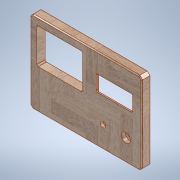
# Autodesk Inventor part: EW_Holzplatte
Saved by Autodesk Inventor 2020 (Build 240168000, 168)
## iProperties
Created: 2020-06-21
Part Number: EW_Holzplatte
Material: Eiche, Rot
Document SubType Name: Modeling
Designer: Johannes
Density: 0.673 g/cm^3
Appearance: Eiche - Fischgrätmuster
Author: Johannes
Autodesk Inventor part; units mm, degrees
ref_plane "YZ Plane" through (0, 0, 0) normal (1, 0, 0) x (0, 1, 0)
ref_plane "XZ Plane" through (0, 0, 0) normal (0, 1, 0) x (-1, 0, 0)
ref_plane "XY Plane" through (0, 0, 0) normal (0, 0, 1) x (1, 0, 0)
sketch "Skizze1" plane through (0, 0, 0) normal (0, 0, 1) x (1, 0, 0)
  line L0 (-122.5, 90) -> (122.5, 90)
  line L1 (122.5, 90) -> (122.5, -90)
  line L2 (122.5, -90) -> (-122.5, -90)
  line L3 (-122.5, -90) -> (-122.5, 90)
  line L4 (-122.5, 90) -> (122.5, -90) construction
  line L5 (122.5, 90) -> (-122.5, -90) construction
  point P0 (0, 0)
  dimension "d0" = 245
  dimension "d1" = 180
  constraints: 12 end point, 2 midpoint, 2 parallel, 1 horizontal, 1 perpendicular
  measures "d0" distance of L1.end L2.end
  measures "d1" distance of L0.end L1.end
extrude "Extrusion1" add sketch "Skizze1" along normal blind 18
sketch "Skizze3" plane through (0, 0, 18) normal (0, 0, 1) x (1, 0, 0)
  line L0 (22.5, 47.5) -> (102.5, 47.5)
  line L1 (102.5, 47.5) -> (102.5, 12.5)
  line L2 (102.5, 12.5) -> (22.5, 12.5)
  line L3 (22.5, 12.5) -> (22.5, 47.5)
  line L4 (22.5, 47.5) -> (102.5, 12.5) construction
  line L5 (102.5, 47.5) -> (22.5, 12.5) construction
  line L6 (122.5, 90) -> (-122.5, 90) projected
  line L7 (122.5, -90) -> (122.5, 90) projected
  point P0 (0, 0)
  point P1 (62.5, 30)
  dimension "d12" = 80
  dimension "d13" = 35
  dimension "d32" = 60
  dimension "d33" = 60
  constraints: 12 end point, 2 midpoint, 2 parallel, 1 horizontal, 1 perpendicular
  measures "d12" distance of L0.start L0.end
  measures "d13" distance of L2.end L0.start
  measures "d32" distance from line of L6 point (62.5, 30)
  measures "d33" distance from line of L7 point (62.5, 30)
extrude "Extrusion2" cut sketch "Skizze3" against normal blind 3
sketch "Skizze4" plane through (0, 0, 0) normal (0, 0, -1) x (-1, 0, 0)
  line L0 (-115, 71.75) -> (-10, 71.75)
  line L1 (-10, 71.75) -> (-10, -25.25)
  line L2 (-10, -25.25) -> (-115, -25.25)
  line L3 (-115, -25.25) -> (-115, 71.75)
  line L4 (-115, 71.75) -> (-10, -25.25) construction
  line L5 (-10, 71.75) -> (-115, -25.25) construction
  line L6 (-122.5, 90) -> (122.5, 90) projected
  line L7 (-122.5, -90) -> (-122.5, 90) projected
  point P0 (0, 0)
  point P1 (-62.5, 23.25)
  dimension "d20" = 60
  dimension "d21" = 105
  dimension "d22" = 97
  dimension "d23" = 18.25
  constraints: 12 end point, 2 midpoint, 2 parallel, 1 horizontal, 1 perpendicular
  measures "d20" distance from line of L7 point (-62.5, 23.25)
  measures "d21" distance of L0.start L0.end
  measures "d22" distance of L2.end L0.start
  measures "d23" distance between parallel lines of L0 L6
extrude "Extrusion3" cut sketch "Skizze4" against normal blind 6
sketch "Skizze5" plane through (0, 0, 6) normal (0, 0, -1) x (-1, 0, 0)
  line L0 (-115, 51) -> (-10, 51)
  line L1 (-10, 51) -> (-10, -5)
  line L2 (-10, -5) -> (-115, -5)
  line L3 (-115, -5) -> (-115, 51)
  line L4 (-115, 51) -> (-10, -5) construction
  line L5 (-10, 51) -> (-115, -5) construction
  line L6 (-122.5, 90) -> (122.5, 90) projected
  line L7 (-122.5, -90) -> (-122.5, 90) projected
  point P0 (0, 0)
  point P1 (-62.5, 23)
  dimension "d26" = 105
  dimension "d34" = 60
  dimension "d35" = 39
  dimension "d36" = 95
  constraints: 12 end point, 2 midpoint, 2 parallel, 1 horizontal, 1 perpendicular
  measures "d26" distance of L0.start L0.end
  measures "d34" distance from line of L7 point (-62.5, 23)
  measures "d35" distance between parallel lines of L6 L0
  measures "d36" distance between parallel lines of L2 L6
extrude "Extrusion4" cut sketch "Skizze5" against normal blind 9
sketch "Skizze7" plane through (0, 0, 0) normal (0, 0, -1) x (-1, 0, 0)
  circle A0 centre (-37.5, -42.5) radius 6
  circle A1 centre (-87.5, -42.5) radius 3.5
  line L0 (-122.5, -90) -> (-122.5, 90) projected
  line L1 (-122.5, 90) -> (122.5, 90) projected
  point P0 (0, 0)
  dimension "d44" = 35
  dimension "d45" = 50
  dimension "d46" = 12
  dimension "d47" = 7
  dimension "d48" = 132.5
  constraints: 2 centre point, 1 horizontal alignment
  measures "d44" distance from line of L0 A1.centre
  measures "d45" distance of A0.centre A1.centre
  measures "d46" diameter of A0
  measures "d47" diameter of A1
  measures "d48" distance from line of L1 A0.centre
extrude "Extrusion6" cut sketch "Skizze7" against normal through all
sketch "Skizze8" plane through (0, 0, 0) normal (0, 0, -1) x (-1, 0, 0)
  line L0 (-45.5, -24.5) -> (-29.5, -24.5)
  line L1 (-29.5, -24.5) -> (-29.5, -60.5)
  line L2 (-29.5, -60.5) -> (-45.5, -60.5)
  line L3 (-45.5, -60.5) -> (-45.5, -24.5)
  line L4 (-45.5, -24.5) -> (-29.5, -60.5) construction
  line L5 (-29.5, -24.5) -> (-45.5, -60.5) construction
  circle A0 centre (-37.5, -42.5) radius 6 projected
  point P0 (0, 0)
  dimension "d51" = 16
  dimension "d52" = 36
  constraints: 12 end point, 3 midpoint, 2 parallel, 1 coincident, 1 horizontal, 1 perpendicular
  measures "d51" distance of L0.start L0.end
  measures "d52" distance of L0.end L1.end
extrude "Extrusion7" cut sketch "Skizze8" against normal blind 12
sketch "Skizze9" plane through (0, 0, 0) normal (0, 0, -1) x (-1, 0, 0)
  line L0 (-93.5, -31.5) -> (-81.5, -31.5)
  line L1 (-81.5, -31.5) -> (-81.5, -53.5)
  line L2 (-81.5, -53.5) -> (-93.5, -53.5)
  line L3 (-93.5, -53.5) -> (-93.5, -31.5)
  circle A0 centre (-87.5, -42.5) radius 3.5 projected
  line L4 (-93.5, -31.5) -> (-81.5, -53.5) construction
  line L5 (-81.5, -31.5) -> (-93.5, -53.5) construction
  point P0 (0, 0)
  dimension "d55" = 12
  dimension "d56" = 22
  constraints: 12 end point, 2 midpoint, 2 parallel, 1 horizontal, 1 perpendicular
  measures "d55" distance of L1.end L2.end
  measures "d56" distance of L0.end L1.end
extrude "Extrusion8" cut sketch "Skizze9" against normal blind 5
sketch "Skizze10" plane through (0, 0, 18) normal (0, 0, 1) x (1, 0, 0)
  circle A0 centre (87.5, -42.5) radius 3.5 projected
  circle A1 centre (87.5, -42.5) radius 10
  point P0 (0, 0)
  dimension "d59" = 20
  constraints: 1 centre point, 1 coincident
  measures "d59" diameter of A1
extrude "Extrusion9" cut sketch "Skizze10" against normal blind 9
sketch "Skizze11" plane through (0, 0, 0) normal (0, 0, -1) x (-1, 0, 0)
  line L0 (7.5, 74) -> (107.5, 74)
  line L1 (107.5, 74) -> (107.5, -3.5)
  line L2 (107.5, -3.5) -> (7.5, -3.5)
  line L3 (7.5, -3.5) -> (7.5, 74)
  line L4 (7.5, 74) -> (107.5, -3.5) construction
  line L5 (107.5, 74) -> (7.5, -3.5) construction
  line L6 (-122.5, 90) -> (122.5, 90) projected
  line L7 (122.5, 90) -> (122.5, -90) projected
  point P0 (0, 0)
  point P1 (57.5, 35.25)
  dimension "d62" = 16
  dimension "d63" = 15
  dimension "d64" = 100
  dimension "d65" = 77.5
  constraints: 12 end point, 2 midpoint, 2 parallel, 1 horizontal, 1 perpendicular
  measures "d62" distance between parallel lines of L6 L0
  measures "d63" distance between parallel lines of L7 L1
  measures "d64" distance of L0.start L0.end
  measures "d65" distance of L0.end L1.end
extrude "Extrusion10" cut sketch "Skizze11" against normal through all
fillet "Rundung1" radius 3 26 edges at (22.5, 47.5, 16.5) (22.5, 12.5, 16.5) (102.5, 12.5, 16.5) (102.5, 47.5, 16.5) (115, 71.75, 3) (10, 71.75, 3) (10, -25.25, 3) (115, -25.25, 3) (115, 51, 10.5) (10, 51, 10.5) (10, -5, 10.5) (115, -5, 10.5) (45.5, -25.25, 3) (29.5, -25.25, 3) (29.5, -24.5, 9) (45.5, -24.5, 9) (45.5, -60.5, 6) (29.5, -60.5, 6) (93.5, -31.5, 2.5) (81.5, -31.5, 2.5) (81.5, -53.5, 2.5) (93.5, -53.5, 2.5) (-7.5, 74, 9) (-7.5, -3.5, 9) (-107.5, -3.5, 9) (-107.5, 74, 9)
chamfer "Fase1" distance 6 angle 45 4 edges at (-122.5, 90, 9) (122.5, 90, 9) (122.5, -90, 9) (-122.5, -90, 9)
chamfer "Fase2" distance 2 angle 45 8 edges at (0, 90, 18) (-119.5, 87, 18) (-122.5, 0, 18) (-119.5, -87, 18) (0, -90, 18) (119.5, -87, 18) (122.5, 0, 18) (119.5, 87, 18)
